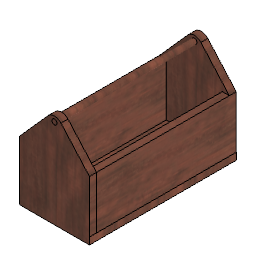
091325_Amanda Tu_Fusion Tutorial (Autodesk Fusion 360 design; units mm, degrees)
part number: 2025-09-13-15-11-52-088
part number: 2025-09-13-15-35-29-478
Autodesk Fusion 360 part; units mm, degrees
sketch "Sketch1" plane through (0, 0, 0) normal (0, 1, 0) x (1, 0, 0)
  line L0 (0, 0) -> (0, -300)
  line L1 (0, -300) -> (400, -300)
  line L2 (0, 0) -> (400, 0)
  line L3 (400, -300) -> (400, 0)
  line L4 (0, -299.8347) -> (200, -299.8347) construction
  line L5 (200, -299.8347) -> (200, -524.8347) construction
  line L6 (162.6417, -482.8374) -> (0, -300)
  line L7 (237.3583, -482.8374) -> (400, -300)
  arc A0 (162.6417, -482.8374) -> (237.3583, -482.8374) centre (200, -449.6056) ccw
  circle A1 centre (200, -470) radius 15
  dimension "d1" = 300
  dimension "d2" = 400
  dimension "d3" = 400
  dimension "d4" = 200
  dimension "d5" = 225
  dimension "d6" = 50
  dimension "d7" = 30
  constraint coincident L0.start L2.start
  constraint vertical L0
  constraint perpendicular L0 L1
  constraint perpendicular L0 L2
  constraint coincident L0 L4.start
  constraint perpendicular L0 L4
  constraint perpendicular L1 L5
  constraint coincident L5.end L6
  constraint coincident L5.end L7
  constraint tangent L6 A0
  constraint tangent L7 A0
  constraint coincident L5 A1.centre
  measures "d1" distance of L0.start L0.end
  measures "d2" distance of L0.end L1.end
  measures "d3" distance of L0.start L2.end
  measures "d4" distance of L4.start L4.end
  measures "d5" distance of L4.end L5.end
  measures "d6" radius of A0
  measures "d7" diameter of A1
extrude "Extrude1" add sketch "Sketch1" along normal blind 40 makes body 1
sketch "Sketch2" plane through (0, 40, 0) normal (0, 1, 0) x (-1, 0, 0)
  circle A0 centre (-200, 470) radius 15
  line L0 (0, 0) -> (0, 300)
  line L1 (0, 300) -> (-162.6417, 482.8374)
  arc A1 (-162.6417, 482.8374) -> (-237.3583, 482.8374) centre (-200, 449.6056) ccw
  line L2 (-237.3583, 482.8374) -> (-400, 300)
  line L3 (-400, 300) -> (-400, 0)
  line L4 (-400, 0) -> (0, 0)
  line L5 (-400, 0) -> (-360, 0)
  line L6 (-360, 0) -> (-360, 300)
  line L7 (-360, 300) -> (-400, 300)
  dimension "d10" = 40
  constraint coincident L3.end L4.start
  constraint perpendicular L3 L5
  constraint perpendicular L4 L6
  constraint coincident L2.end L3.start
  constraint perpendicular L3 L7
  measures "d10" distance of L3.end L5.end
extrude "Extrude1'" add sketch "Sketch2" along normal blind 800 separate body contours L3 L4 L5 L6 L7 makes body 2 in component "Component"
copy_body "CopyPasteBodies1" bodies 2 makes body 3
move_body "Move1" bodies 3 to x (1, 0, 0) y (0, 1, 0) z (0, 0, 1) at (0, 0, 0)
copy_body "CopyPasteBodies2" bodies 3 makes body 4
move_body "Move2" bodies 4 to x (1, 0, 0) y (0, 1, 0) z (0, 0, 1) at (-360, 0, 0)
copy_body "CopyPasteBodies3" bodies 1 makes body 5
move_body "Move3" bodies 5 to x (1, 0, 0) y (0, 1, 0) z (0, 0, 1) at (0, 800, 0)
sketch "Sketch4" plane through (0, 0, 0) normal (0, 0, 1) x (1, 0, 0)
  line L0 (399.9616, 841.1257) -> (0, 841.1257)
  line L1 (0, 841.1257) -> (0, 0)
  line L2 (0, 0) -> (399.9616, 0)
  line L3 (399.9616, 0) -> (399.9616, 841.1257)
  constraint horizontal L0
  constraint vertical L1
  constraint horizontal L2
  constraint vertical L3
  constraint coincident L1.end L2.start
extrude "Extrude2" add sketch "Sketch4" against normal blind 40 bodies 1 3 4 5
sketch "Sketch5" plane through (0, 0, 0) normal (0, 1, 0) x (1, 0, 0)
sketch "Sketch6" plane through (0, 0, 0) normal (0, 1, 0) x (1, 0, 0)
  circle A0 centre (200.0265, -470.4475) radius 15
  dimension "d15" = 30
  measures "d15" diameter of A0
sketch "Sketch7" plane through (0, 0, 0) normal (0, 1, 0) x (1, 0, 0)
extrude "Extrude3" add sketch "Sketch6" along normal blind 840 separate body makes body 6
component "Component" placed x (1, 0, 0) y (0, 1, 0) z (0, 0, 1) at (0, 0, 0)
